Autodesk Fusion 360 part; units mm, degrees
(part 6 of 7)
extrude "v21 socket head clearance (2)" cut sketch "v21 socket head clearance profile (2)" against normal blind 3.22 bodies 1 in component "01 Front optical bezel"
ref_plane "WorkPlane88" through (0, 0, -9.48) normal (0, 0, 1) x (1, 0, 0) in component "05 Rear electronics housing"
sketch "v21 closure blind clearance profile (2)" plane through (0, 0, -9.48) normal (0, 0, 1) x (1, 0, 0) in component "05 Rear electronics housing"
  circle A0 centre (6, 54) radius 1.8
  dimension "d1678" = 3.6
  measures "d1678" diameter of A0
extrude "v21 closure blind clearance (2)" cut sketch "v21 closure blind clearance profile (2)" against normal blind 19.72 bodies 66 in component "05 Rear electronics housing"
ref_plane "WorkPlane67" through (0, 0, 0.02) normal (0, 0, 1) x (1, 0, 0) in component "01 Front optical bezel"
sketch "v21 closure screw clearance profile (3)" plane through (0, 0, 0.02) normal (0, 0, 1) x (1, 0, 0) in component "01 Front optical bezel"
  circle A0 centre (96, 54) radius 1.8
  dimension "d1683" = 3.6
  measures "d1683" diameter of A0
extrude "v21 closure screw clearance (3)" cut sketch "v21 closure screw clearance profile (3)" against normal blind 9.6 bodies 1 in component "01 Front optical bezel"
ref_plane "WorkPlane68" through (0, 0, 0.02) normal (0, 0, 1) x (1, 0, 0) in component "01 Front optical bezel"
sketch "v21 socket head clearance profile (3)" plane through (0, 0, 0.02) normal (0, 0, 1) x (1, 0, 0) in component "01 Front optical bezel"
  circle A0 centre (96, 54) radius 3.4
  dimension "d1688" = 6.8
  measures "d1688" diameter of A0
extrude "v21 socket head clearance (3)" cut sketch "v21 socket head clearance profile (3)" against normal blind 3.22 bodies 1 in component "01 Front optical bezel"
ref_plane "WorkPlane89" through (0, 0, -9.48) normal (0, 0, 1) x (1, 0, 0) in component "05 Rear electronics housing"
sketch "v21 closure blind clearance profile (3)" plane through (0, 0, -9.48) normal (0, 0, 1) x (1, 0, 0) in component "05 Rear electronics housing"
  circle A0 centre (96, 54) radius 1.8
  dimension "d1693" = 3.6
  measures "d1693" diameter of A0
extrude "v21 closure blind clearance (3)" cut sketch "v21 closure blind clearance profile (3)" against normal blind 19.72 bodies 66 in component "05 Rear electronics housing"
ref_plane "WorkPlane69" through (0, 0, -2.6) normal (0, 0, 1) x (1, 0, 0) in component "01 Front optical bezel"
sketch "v21 optical blind clearance profile" plane through (0, 0, -2.6) normal (0, 0, 1) x (1, 0, 0) in component "01 Front optical bezel"
  circle A0 centre (60, 6) radius 1.8
  dimension "d1698" = 3.6
  measures "d1698" diameter of A0
extrude "v21 optical blind clearance" cut sketch "v21 optical blind clearance profile" against normal blind 4.9 bodies 1 in component "01 Front optical bezel"
ref_plane "WorkPlane15" through (0, 0, -7.45) normal (0, 0, 1) x (1, 0, 0) in component "04 Optical retainer"
sketch "v21 optical screw clearance profile" plane through (0, 0, -7.45) normal (0, 0, 1) x (1, 0, 0) in component "04 Optical retainer"
  circle A0 centre (60, 6) radius 1.8
  dimension "d1703" = 3.6
  measures "d1703" diameter of A0
extrude "v21 optical screw clearance" cut sketch "v21 optical screw clearance profile" against normal blind 1.65 bodies 53 in component "04 Optical retainer"
ref_plane "WorkPlane70" through (0, 0, -2.6) normal (0, 0, 1) x (1, 0, 0) in component "01 Front optical bezel"
sketch "v21 optical blind clearance profile (1)" plane through (0, 0, -2.6) normal (0, 0, 1) x (1, 0, 0) in component "01 Front optical bezel"
  circle A0 centre (60, 54) radius 1.8
  dimension "d1708" = 3.6
  measures "d1708" diameter of A0
extrude "v21 optical blind clearance (1)" cut sketch "v21 optical blind clearance profile (1)" against normal blind 4.9 bodies 1 in component "01 Front optical bezel"
ref_plane "WorkPlane16" through (0, 0, -7.45) normal (0, 0, 1) x (1, 0, 0) in component "04 Optical retainer"
sketch "v21 optical screw clearance profile (1)" plane through (0, 0, -7.45) normal (0, 0, 1) x (1, 0, 0) in component "04 Optical retainer"
  circle A0 centre (60, 54) radius 1.8
  dimension "d1713" = 3.6
  measures "d1713" diameter of A0
extrude "v21 optical screw clearance (1)" cut sketch "v21 optical screw clearance profile (1)" against normal blind 1.65 bodies 53 in component "04 Optical retainer"
ref_plane "WorkPlane90" through (0, 0, -11.38) normal (0, 0, 1) x (1, 0, 0) in component "05 Rear electronics housing"
sketch "v21 yoke blind clearance profile" plane through (0, 0, -11.38) normal (0, 0, 1) x (1, 0, 0) in component "05 Rear electronics housing"
  circle A0 centre (35, 38) radius 1.8
  dimension "d1718" = 3.6
  measures "d1718" diameter of A0
extrude "v21 yoke blind clearance" cut sketch "v21 yoke blind clearance profile" against normal blind 6.82 bodies 66 in component "05 Rear electronics housing"
ref_plane "WorkPlane42" through (0, 0, -9.38) normal (0, 0, 1) x (1, 0, 0) in component "06 Electronics retaining yoke"
sketch "v21 yoke screw clearance profile" plane through (0, 0, -9.38) normal (0, 0, 1) x (1, 0, 0) in component "06 Electronics retaining yoke"
  circle A0 centre (35, 38) radius 1.8
  dimension "d1723" = 3.6
  measures "d1723" diameter of A0
extrude "v21 yoke screw clearance" cut sketch "v21 yoke screw clearance profile" against normal blind 2.04 bodies 106 in component "06 Electronics retaining yoke"
ref_plane "WorkPlane91" through (0, 0, -11.38) normal (0, 0, 1) x (1, 0, 0) in component "05 Rear electronics housing"
sketch "v21 yoke blind clearance profile (1)" plane through (0, 0, -11.38) normal (0, 0, 1) x (1, 0, 0) in component "05 Rear electronics housing"
  circle A0 centre (103, 38) radius 1.8
  dimension "d1728" = 3.6
  measures "d1728" diameter of A0
extrude "v21 yoke blind clearance (1)" cut sketch "v21 yoke blind clearance profile (1)" against normal blind 6.82 bodies 66 in component "05 Rear electronics housing"
ref_plane "WorkPlane43" through (0, 0, -9.38) normal (0, 0, 1) x (1, 0, 0) in component "06 Electronics retaining yoke"
sketch "v21 yoke screw clearance profile (1)" plane through (0, 0, -9.38) normal (0, 0, 1) x (1, 0, 0) in component "06 Electronics retaining yoke"
  circle A0 centre (103, 38) radius 1.8
  dimension "d1733" = 3.6
  measures "d1733" diameter of A0
extrude "v21 yoke screw clearance (1)" cut sketch "v21 yoke screw clearance profile (1)" against normal blind 2.04 bodies 106 in component "06 Electronics retaining yoke"
ref_plane "WorkPlane44" through (0, 0, -22.85) normal (0, 0, 1) x (1, 0, 0) in component "06 Electronics retaining yoke"
sketch "v21 PCB axial clearance profile" plane through (0, 0, -22.85) normal (0, 0, 1) x (1, 0, 0) in component "06 Electronics retaining yoke"
  line L0 (13.09, 33.99) -> (15.11, 33.99)
  line L1 (15.11, 33.99) -> (15.11, 36.01)
  line L2 (15.11, 36.01) -> (13.09, 36.01)
  line L3 (13.09, 36.01) -> (13.09, 33.99)
  dimension "d1738" = 2.02
  dimension "d1739" = 2.02
  measures "d1738" horizontal distance of L0.start L0.end
  measures "d1739" vertical distance of L0.end L1.end
extrude "v21 PCB axial clearance" cut sketch "v21 PCB axial clearance profile" against normal blind 0.22 bodies 106 in component "06 Electronics retaining yoke"
ref_plane "WorkPlane45" through (0, 0, -22.85) normal (0, 0, 1) x (1, 0, 0) in component "06 Electronics retaining yoke"
sketch "v21 PCB axial clearance profile (1)" plane through (0, 0, -22.85) normal (0, 0, 1) x (1, 0, 0) in component "06 Electronics retaining yoke"
  line L0 (13.09, 50.99) -> (15.11, 50.99)
  line L1 (15.11, 50.99) -> (15.11, 53.01)
  line L2 (15.11, 53.01) -> (13.09, 53.01)
  line L3 (13.09, 53.01) -> (13.09, 50.99)
  dimension "d1744" = 2.02
  dimension "d1745" = 2.02
  measures "d1744" horizontal distance of L0.start L0.end
  measures "d1745" vertical distance of L0.end L1.end
extrude "v21 PCB axial clearance (1)" cut sketch "v21 PCB axial clearance profile (1)" against normal blind 0.22 bodies 106 in component "06 Electronics retaining yoke"
ref_plane "WorkPlane46" through (0, 0, -22.85) normal (0, 0, 1) x (1, 0, 0) in component "06 Electronics retaining yoke"
sketch "v21 PCB axial clearance profile (2)" plane through (0, 0, -22.85) normal (0, 0, 1) x (1, 0, 0) in component "06 Electronics retaining yoke"
  line L0 (26.89, 33.99) -> (28.91, 33.99)
  line L1 (28.91, 33.99) -> (28.91, 36.01)
  line L2 (28.91, 36.01) -> (26.89, 36.01)
  line L3 (26.89, 36.01) -> (26.89, 33.99)
  dimension "d1750" = 2.02
  dimension "d1751" = 2.02
  measures "d1750" horizontal distance of L0.start L0.end
  measures "d1751" vertical distance of L0.end L1.end
extrude "v21 PCB axial clearance (2)" cut sketch "v21 PCB axial clearance profile (2)" against normal blind 0.22 bodies 106 in component "06 Electronics retaining yoke"
ref_plane "WorkPlane47" through (0, 0, -22.85) normal (0, 0, 1) x (1, 0, 0) in component "06 Electronics retaining yoke"
sketch "v21 PCB axial clearance profile (3)" plane through (0, 0, -22.85) normal (0, 0, 1) x (1, 0, 0) in component "06 Electronics retaining yoke"
  line L0 (26.89, 50.99) -> (28.91, 50.99)
  line L1 (28.91, 50.99) -> (28.91, 53.01)
  line L2 (28.91, 53.01) -> (26.89, 53.01)
  line L3 (26.89, 53.01) -> (26.89, 50.99)
  dimension "d1756" = 2.02
  dimension "d1757" = 2.02
  measures "d1756" horizontal distance of L0.start L0.end
  measures "d1757" vertical distance of L0.end L1.end
extrude "v21 PCB axial clearance (3)" cut sketch "v21 PCB axial clearance profile (3)" against normal blind 0.22 bodies 106 in component "06 Electronics retaining yoke"
ref_plane "WorkPlane48" through (0, 0, -19.65) normal (0, 0, 1) x (1, 0, 0) in component "06 Electronics retaining yoke"
sketch "v21 DPDT axial clearance profile" plane through (0, 0, -19.65) normal (0, 0, 1) x (1, 0, 0) in component "06 Electronics retaining yoke"
  line L0 (55.89, 49.69) -> (56.91, 49.69)
  line L1 (56.91, 49.69) -> (56.91, 52.01)
  line L2 (56.91, 52.01) -> (55.89, 52.01)
  line L3 (55.89, 52.01) -> (55.89, 49.69)
  dimension "d1762" = 1.02
  dimension "d1763" = 2.32
  measures "d1762" horizontal distance of L0.start L0.end
  measures "d1763" vertical distance of L0.end L1.end
extrude "v21 DPDT axial clearance" cut sketch "v21 DPDT axial clearance profile" against normal blind 0.22 bodies 106 in component "06 Electronics retaining yoke"
ref_plane "WorkPlane49" through (0, 0, -19.65) normal (0, 0, 1) x (1, 0, 0) in component "06 Electronics retaining yoke"
sketch "v21 DPDT axial clearance profile (1)" plane through (0, 0, -19.65) normal (0, 0, 1) x (1, 0, 0) in component "06 Electronics retaining yoke"
  line L0 (63.09, 49.69) -> (64.11, 49.69)
  line L1 (64.11, 49.69) -> (64.11, 52.01)
  line L2 (64.11, 52.01) -> (63.09, 52.01)
  line L3 (63.09, 52.01) -> (63.09, 49.69)
  dimension "d1768" = 1.02
  dimension "d1769" = 2.32
  measures "d1768" horizontal distance of L0.start L0.end
  measures "d1769" vertical distance of L0.end L1.end
extrude "v21 DPDT axial clearance (1)" cut sketch "v21 DPDT axial clearance profile (1)" against normal blind 0.22 bodies 106 in component "06 Electronics retaining yoke"
ref_plane "WorkPlane50" through (0, 0, -11.2) normal (0, 0, 1) x (1, 0, 0) in component "06 Electronics retaining yoke"
sketch "v21 XIAO axial clearance profile" plane through (0, 0, -11.2) normal (0, 0, 1) x (1, 0, 0) in component "06 Electronics retaining yoke"
  line L0 (110.8, 35.4) -> (112.1, 35.4)
  line L1 (112.1, 35.4) -> (112.1, 56.6)
  line L2 (112.1, 56.6) -> (110.8, 56.6)
  line L3 (110.8, 56.6) -> (110.8, 35.4)
  dimension "d1774" = 1.3
  dimension "d1775" = 21.2
  measures "d1774" horizontal distance of L0.start L0.end
  measures "d1775" vertical distance of L0.end L1.end
extrude "v21 XIAO axial clearance" cut sketch "v21 XIAO axial clearance profile" against normal blind 0.25 bodies 106 in component "06 Electronics retaining yoke"
ref_plane "WorkPlane17" through (0, 0, -7.47) normal (0, 0, 1) x (1, 0, 0) in component "04 Optical retainer"
sketch "v21 optical stack allowance profile" plane through (0, 0, -7.47) normal (0, 0, 1) x (1, 0, 0) in component "04 Optical retainer"
  line L0 (7.99, 10.99) -> (112.01, 10.99)
  line L1 (112.01, 10.99) -> (112.01, 49.01)
  line L2 (112.01, 49.01) -> (7.99, 49.01)
  line L3 (7.99, 49.01) -> (7.99, 10.99)
  dimension "d1780" = 104.02
  dimension "d1781" = 38.02
  measures "d1780" horizontal distance of L0.start L0.end
  measures "d1781" vertical distance of L0.end L1.end
extrude "v21 optical stack allowance" cut sketch "v21 optical stack allowance profile" against normal blind 0.255 bodies 53 in component "04 Optical retainer"
ref_plane "WorkPlane18" through (0, 0, -4.34) normal (0, 0, 1) x (1, 0, 0) in component "04 Optical retainer"
sketch "v21 LED cushion clearance profile" plane through (0, 0, -4.34) normal (0, 0, 1) x (1, 0, 0) in component "04 Optical retainer"
  line L0 (38.49, 5.19) -> (41.51, 5.19)
  line L1 (41.51, 5.19) -> (41.51, 10.81)
  line L2 (41.51, 10.81) -> (38.49, 10.81)
  line L3 (38.49, 10.81) -> (38.49, 5.19)
  dimension "d1786" = 3.02
  dimension "d1787" = 5.62
  measures "d1786" horizontal distance of L0.start L0.end
  measures "d1787" vertical distance of L0.end L1.end
extrude "v21 LED cushion clearance" cut sketch "v21 LED cushion clearance profile" against normal blind 0.26 bodies 53 in component "04 Optical retainer"
ref_plane "WorkPlane19" through (0, 0, -4.34) normal (0, 0, 1) x (1, 0, 0) in component "04 Optical retainer"
sketch "v21 LED cushion clearance profile (1)" plane through (0, 0, -4.34) normal (0, 0, 1) x (1, 0, 0) in component "04 Optical retainer"
  line L0 (38.49, 49.19) -> (41.51, 49.19)
  line L1 (41.51, 49.19) -> (41.51, 54.81)
  line L2 (41.51, 54.81) -> (38.49, 54.81)
  line L3 (38.49, 54.81) -> (38.49, 49.19)
  dimension "d1792" = 3.02
  dimension "d1793" = 5.62
  measures "d1792" horizontal distance of L0.start L0.end
  measures "d1793" vertical distance of L0.end L1.end
extrude "v21 LED cushion clearance (1)" cut sketch "v21 LED cushion clearance profile (1)" against normal blind 0.26 bodies 53 in component "04 Optical retainer"
ref_plane "WorkPlane20" through (0, 0, -4.34) normal (0, 0, 1) x (1, 0, 0) in component "04 Optical retainer"
sketch "v21 LED cushion clearance profile (2)" plane through (0, 0, -4.34) normal (0, 0, 1) x (1, 0, 0) in component "04 Optical retainer"
  line L0 (78.49, 5.19) -> (81.51, 5.19)
  line L1 (81.51, 5.19) -> (81.51, 10.81)
  line L2 (81.51, 10.81) -> (78.49, 10.81)
  line L3 (78.49, 10.81) -> (78.49, 5.19)
  dimension "d1798" = 3.02
  dimension "d1799" = 5.62
  measures "d1798" horizontal distance of L0.start L0.end
  measures "d1799" vertical distance of L0.end L1.end
extrude "v21 LED cushion clearance (2)" cut sketch "v21 LED cushion clearance profile (2)" against normal blind 0.26 bodies 53 in component "04 Optical retainer"
ref_plane "WorkPlane21" through (0, 0, -4.34) normal (0, 0, 1) x (1, 0, 0) in component "04 Optical retainer"
sketch "v21 LED cushion clearance profile (3)" plane through (0, 0, -4.34) normal (0, 0, 1) x (1, 0, 0) in component "04 Optical retainer"
  line L0 (78.49, 49.19) -> (81.51, 49.19)
  line L1 (81.51, 49.19) -> (81.51, 54.81)
  line L2 (81.51, 54.81) -> (78.49, 54.81)
  line L3 (78.49, 54.81) -> (78.49, 49.19)
  dimension "d1804" = 3.02
  dimension "d1805" = 5.62
  measures "d1804" horizontal distance of L0.start L0.end
  measures "d1805" vertical distance of L0.end L1.end
extrude "v21 LED cushion clearance (3)" cut sketch "v21 LED cushion clearance profile (3)" against normal blind 0.26 bodies 53 in component "04 Optical retainer"
ref_plane "WorkPlane71" through (0, 0, -2.4) normal (0, 0, 1) x (1, 0, 0) in component "01 Front optical bezel"
sketch "v21 LED solder-wire exit profile" plane through (0, 0, -2.4) normal (0, 0, 1) x (1, 0, 0) in component "01 Front optical bezel"
  line L0 (34.4, 4.8) -> (35.9, 4.8)
  line L1 (35.9, 4.8) -> (35.9, 8.8)
  line L2 (35.9, 8.8) -> (34.4, 8.8)
  line L3 (34.4, 8.8) -> (34.4, 4.8)
  dimension "d1810" = 1.5
  dimension "d1811" = 4
  measures "d1810" horizontal distance of L0.start L0.end
  measures "d1811" vertical distance of L0.end L1.end
extrude "v21 LED solder-wire exit" cut sketch "v21 LED solder-wire exit profile" against normal blind 2.2 bodies 1 in component "01 Front optical bezel"
ref_plane "WorkPlane72" through (0, 0, -2.4) normal (0, 0, 1) x (1, 0, 0) in component "01 Front optical bezel"
sketch "v21 LED solder-wire exit profile (1)" plane through (0, 0, -2.4) normal (0, 0, 1) x (1, 0, 0) in component "01 Front optical bezel"
  line L0 (44.1, 4.8) -> (45.6, 4.8)
  line L1 (45.6, 4.8) -> (45.6, 8.8)
  line L2 (45.6, 8.8) -> (44.1, 8.8)
  line L3 (44.1, 8.8) -> (44.1, 4.8)
  dimension "d1816" = 1.5
  dimension "d1817" = 4
  measures "d1816" horizontal distance of L0.start L0.end
  measures "d1817" vertical distance of L0.end L1.end
extrude "v21 LED solder-wire exit (1)" cut sketch "v21 LED solder-wire exit profile (1)" against normal blind 2.2 bodies 1 in component "01 Front optical bezel"
ref_plane "WorkPlane73" through (0, 0, -2.4) normal (0, 0, 1) x (1, 0, 0) in component "01 Front optical bezel"
sketch "v21 LED solder-wire exit profile (2)" plane through (0, 0, -2.4) normal (0, 0, 1) x (1, 0, 0) in component "01 Front optical bezel"
  line L0 (34.4, 51.2) -> (35.9, 51.2)
  line L1 (35.9, 51.2) -> (35.9, 55.2)
  line L2 (35.9, 55.2) -> (34.4, 55.2)
  line L3 (34.4, 55.2) -> (34.4, 51.2)
  dimension "d1822" = 1.5
  dimension "d1823" = 4
  measures "d1822" horizontal distance of L0.start L0.end
  measures "d1823" vertical distance of L0.end L1.end
extrude "v21 LED solder-wire exit (2)" cut sketch "v21 LED solder-wire exit profile (2)" against normal blind 2.2 bodies 1 in component "01 Front optical bezel"
ref_plane "WorkPlane74" through (0, 0, -2.4) normal (0, 0, 1) x (1, 0, 0) in component "01 Front optical bezel"
sketch "v21 LED solder-wire exit profile (3)" plane through (0, 0, -2.4) normal (0, 0, 1) x (1, 0, 0) in component "01 Front optical bezel"
  line L0 (44.1, 51.2) -> (45.6, 51.2)
  line L1 (45.6, 51.2) -> (45.6, 55.2)
  line L2 (45.6, 55.2) -> (44.1, 55.2)
  line L3 (44.1, 55.2) -> (44.1, 51.2)
  dimension "d1828" = 1.5
  dimension "d1829" = 4
  measures "d1828" horizontal distance of L0.start L0.end
  measures "d1829" vertical distance of L0.end L1.end
extrude "v21 LED solder-wire exit (3)" cut sketch "v21 LED solder-wire exit profile (3)" against normal blind 2.2 bodies 1 in component "01 Front optical bezel"
ref_plane "WorkPlane75" through (0, 0, -2.4) normal (0, 0, 1) x (1, 0, 0) in component "01 Front optical bezel"
sketch "v21 LED solder-wire exit profile (4)" plane through (0, 0, -2.4) normal (0, 0, 1) x (1, 0, 0) in component "01 Front optical bezel"
  line L0 (74.4, 4.8) -> (75.9, 4.8)
  line L1 (75.9, 4.8) -> (75.9, 8.8)
  line L2 (75.9, 8.8) -> (74.4, 8.8)
  line L3 (74.4, 8.8) -> (74.4, 4.8)
  dimension "d1834" = 1.5
  dimension "d1835" = 4
  measures "d1834" horizontal distance of L0.start L0.end
  measures "d1835" vertical distance of L0.end L1.end
extrude "v21 LED solder-wire exit (4)" cut sketch "v21 LED solder-wire exit profile (4)" against normal blind 2.2 bodies 1 in component "01 Front optical bezel"
ref_plane "WorkPlane76" through (0, 0, -2.4) normal (0, 0, 1) x (1, 0, 0) in component "01 Front optical bezel"
sketch "v21 LED solder-wire exit profile (5)" plane through (0, 0, -2.4) normal (0, 0, 1) x (1, 0, 0) in component "01 Front optical bezel"
  line L0 (84.1, 4.8) -> (85.6, 4.8)
  line L1 (85.6, 4.8) -> (85.6, 8.8)
  line L2 (85.6, 8.8) -> (84.1, 8.8)
  line L3 (84.1, 8.8) -> (84.1, 4.8)
  dimension "d1840" = 1.5
  dimension "d1841" = 4
  measures "d1840" horizontal distance of L0.start L0.end
  measures "d1841" vertical distance of L0.end L1.end
extrude "v21 LED solder-wire exit (5)" cut sketch "v21 LED solder-wire exit profile (5)" against normal blind 2.2 bodies 1 in component "01 Front optical bezel"
ref_plane "WorkPlane77" through (0, 0, -2.4) normal (0, 0, 1) x (1, 0, 0) in component "01 Front optical bezel"
sketch "v21 LED solder-wire exit profile (6)" plane through (0, 0, -2.4) normal (0, 0, 1) x (1, 0, 0) in component "01 Front optical bezel"
  line L0 (74.4, 51.2) -> (75.9, 51.2)
  line L1 (75.9, 51.2) -> (75.9, 55.2)
  line L2 (75.9, 55.2) -> (74.4, 55.2)
  line L3 (74.4, 55.2) -> (74.4, 51.2)
  dimension "d1846" = 1.5
  dimension "d1847" = 4
  measures "d1846" horizontal distance of L0.start L0.end
  measures "d1847" vertical distance of L0.end L1.end
extrude "v21 LED solder-wire exit (6)" cut sketch "v21 LED solder-wire exit profile (6)" against normal blind 2.2 bodies 1 in component "01 Front optical bezel"
ref_plane "WorkPlane78" through (0, 0, -2.4) normal (0, 0, 1) x (1, 0, 0) in component "01 Front optical bezel"
sketch "v21 LED solder-wire exit profile (7)" plane through (0, 0, -2.4) normal (0, 0, 1) x (1, 0, 0) in component "01 Front optical bezel"
  line L0 (84.1, 51.2) -> (85.6, 51.2)
  line L1 (85.6, 51.2) -> (85.6, 55.2)
  line L2 (85.6, 55.2) -> (84.1, 55.2)
  line L3 (84.1, 55.2) -> (84.1, 51.2)
  dimension "d1852" = 1.5
  dimension "d1853" = 4
  measures "d1852" horizontal distance of L0.start L0.end
  measures "d1853" vertical distance of L0.end L1.end
extrude "v21 LED solder-wire exit (7)" cut sketch "v21 LED solder-wire exit profile (7)" against normal blind 2.2 bodies 1 in component "01 Front optical bezel"
ref_plane "WorkPlane8" through (0, 0, -18) normal (0, 0, 1) x (1, 0, 0) in component "08 Captive RUN PROGRAM slider"
sketch "v21 actuator running clearance profile" plane through (0, 0, -18) normal (0, 0, 1) x (1, 0, 0) in component "08 Captive RUN PROGRAM slider"
  line L0 (58.95, 52.3) -> (61.05, 52.3)
  line L1 (61.05, 52.3) -> (61.05, 54.53)
  line L2 (61.05, 54.53) -> (58.95, 54.53)
  line L3 (58.95, 54.53) -> (58.95, 52.3)
  dimension "d1858" = 2.1
  dimension "d1859" = 2.23
  measures "d1858" horizontal distance of L0.start L0.end
  measures "d1859" vertical distance of L0.end L1.end
extrude "v21 actuator running clearance" cut sketch "v21 actuator running clearance profile" against normal blind 4.6 bodies 131 in component "08 Captive RUN PROGRAM slider"
ref_plane "WorkPlane92" through (0, 0, -13.6) normal (0, 0, 1) x (1, 0, 0) in component "05 Rear electronics housing"
sketch "v21 reset guide running clearance profile" plane through (0, 0, -13.6) normal (0, 0, 1) x (1, 0, 0) in component "05 Rear electronics housing"
  line L0 (116.1, 52.45) -> (120.2, 52.45)
  line L1 (120.2, 52.45) -> (120.2, 56.95)
  line L2 (120.2, 56.95) -> (116.1, 56.95)
  line L3 (116.1, 56.95) -> (116.1, 52.45)
  dimension "d1864" = 4.1
  dimension "d1865" = 4.5
  measures "d1864" horizontal distance of L0.start L0.end
  measures "d1865" vertical distance of L0.end L1.end
extrude "v21 reset guide running clearance" cut sketch "v21 reset guide running clearance profile" against normal blind 3.1 bodies 66 in component "05 Rear electronics housing"
ref_plane "WorkPlane51" through (0, 0, -13.6) normal (0, 0, 1) x (1, 0, 0) in component "06 Electronics retaining yoke"
sketch "v21 reset roof running clearance profile" plane through (0, 0, -13.6) normal (0, 0, 1) x (1, 0, 0) in component "06 Electronics retaining yoke"
  line L0 (116.19, 52.79) -> (119.76, 52.79)
  line L1 (119.76, 52.79) -> (119.76, 56.61)
  line L2 (119.76, 56.61) -> (116.19, 56.61)
  line L3 (116.19, 56.61) -> (116.19, 52.79)
  dimension "d1870" = 3.57
  dimension "d1871" = 3.82
  measures "d1870" horizontal distance of L0.start L0.end
  measures "d1871" vertical distance of L0.end L1.end
extrude "v21 reset roof running clearance" cut sketch "v21 reset roof running clearance profile" against normal blind 0.12 bodies 106 in component "06 Electronics retaining yoke"
ref_plane "WorkPlane93" through (0, 0, -29.5) normal (0, 0, 1) x (1, 0, 0) in component "05 Rear electronics housing"
sketch "BOOST insulating landing profile" plane through (0, 0, -29.5) normal (0, 0, 1) x (1, 0, 0) in component "05 Rear electronics housing"
  line L0 (37, 41.5) -> (52.3, 41.5)
  line L1 (52.3, 41.5) -> (52.3, 52.5)
  line L2 (52.3, 52.5) -> (37, 52.5)
  line L3 (37, 52.5) -> (37, 41.5)
  dimension "d1876" = 15.3
  dimension "d1877" = 11
  measures "d1876" horizontal distance of L0.start L0.end
  measures "d1877" vertical distance of L0.end L1.end
extrude "BOOST insulating landing" add sketch "BOOST insulating landing profile" against normal blind 2.2 separate body makes body 197 in component "05 Rear electronics housing"
ref_plane "WorkPlane94" through (0, 0, -27.5) normal (0, 0, 1) x (1, 0, 0) in component "05 Rear electronics housing"
sketch "BOOST lateral locating fence profile" plane through (0, 0, -27.5) normal (0, 0, 1) x (1, 0, 0) in component "05 Rear electronics housing"
  line L0 (36.1, 41.5) -> (37.3, 41.5)
  line L1 (37.3, 41.5) -> (37.3, 52.5)
  line L2 (37.3, 52.5) -> (36.1, 52.5)
  line L3 (36.1, 52.5) -> (36.1, 41.5)
  dimension "d1882" = 1.2
  dimension "d1883" = 11
  measures "d1882" horizontal distance of L0.start L0.end
  measures "d1883" vertical distance of L0.end L1.end
extrude "BOOST lateral locating fence" add sketch "BOOST lateral locating fence profile" against normal blind 4.2 separate body makes body 198 in component "05 Rear electronics housing"
ref_plane "WorkPlane95" through (0, 0, -27.5) normal (0, 0, 1) x (1, 0, 0) in component "05 Rear electronics housing"
sketch "BOOST lateral locating fence profile (1)" plane through (0, 0, -27.5) normal (0, 0, 1) x (1, 0, 0) in component "05 Rear electronics housing"
  line L0 (52, 41.5) -> (53.2, 41.5)
  line L1 (53.2, 41.5) -> (53.2, 52.5)
  line L2 (53.2, 52.5) -> (52, 52.5)
  line L3 (52, 52.5) -> (52, 41.5)
  dimension "d1888" = 1.2
  dimension "d1889" = 11
  measures "d1888" horizontal distance of L0.start L0.end
  measures "d1889" vertical distance of L0.end L1.end
extrude "BOOST lateral locating fence (1)" add sketch "BOOST lateral locating fence profile (1)" against normal blind 4.2 separate body makes body 199 in component "05 Rear electronics housing"
ref_plane "WorkPlane96" through (0, 0, -29.5) normal (0, 0, 1) x (1, 0, 0) in component "05 Rear electronics housing"
sketch "SIGNAL insulating landing profile" plane through (0, 0, -29.5) normal (0, 0, 1) x (1, 0, 0) in component "05 Rear electronics housing"
  line L0 (71, 41) -> (90.5, 41)
  line L1 (90.5, 41) -> (90.5, 53.5)
  line L2 (90.5, 53.5) -> (71, 53.5)
  line L3 (71, 53.5) -> (71, 41)
  dimension "d1894" = 19.5
  dimension "d1895" = 12.5
  measures "d1894" horizontal distance of L0.start L0.end
  measures "d1895" vertical distance of L0.end L1.end
extrude "SIGNAL insulating landing" add sketch "SIGNAL insulating landing profile" against normal blind 2.2 separate body makes body 200 in component "05 Rear electronics housing"
ref_plane "WorkPlane97" through (0, 0, -27.5) normal (0, 0, 1) x (1, 0, 0) in component "05 Rear electronics housing"
sketch "SIGNAL lateral locating fence profile" plane through (0, 0, -27.5) normal (0, 0, 1) x (1, 0, 0) in component "05 Rear electronics housing"
  line L0 (70.1, 41) -> (71.3, 41)
  line L1 (71.3, 41) -> (71.3, 53.5)
  line L2 (71.3, 53.5) -> (70.1, 53.5)
  line L3 (70.1, 53.5) -> (70.1, 41)
  dimension "d1900" = 1.2
  dimension "d1901" = 12.5
  measures "d1900" horizontal distance of L0.start L0.end
  measures "d1901" vertical distance of L0.end L1.end
extrude "SIGNAL lateral locating fence" add sketch "SIGNAL lateral locating fence profile" against normal blind 4.2 separate body makes body 201 in component "05 Rear electronics housing"
ref_plane "WorkPlane98" through (0, 0, -27.5) normal (0, 0, 1) x (1, 0, 0) in component "05 Rear electronics housing"
sketch "SIGNAL lateral locating fence profile (1)" plane through (0, 0, -27.5) normal (0, 0, 1) x (1, 0, 0) in component "05 Rear electronics housing"
  line L0 (90.2, 41) -> (91.4, 41)
  line L1 (91.4, 41) -> (91.4, 53.5)
  line L2 (91.4, 53.5) -> (90.2, 53.5)
  line L3 (90.2, 53.5) -> (90.2, 41)
  dimension "d1906" = 1.2
  dimension "d1907" = 12.5
  measures "d1906" horizontal distance of L0.start L0.end
  measures "d1907" vertical distance of L0.end L1.end
extrude "SIGNAL lateral locating fence (1)" add sketch "SIGNAL lateral locating fence profile (1)" against normal blind 4.2 separate body makes body 202 in component "05 Rear electronics housing"
ref_plane "WorkPlane99" through (0, 0, -22) normal (0, 0, 1) x (1, 0, 0) in component "05 Rear electronics housing"
sketch "Harness strap anchor profile" plane through (0, 0, -22) normal (0, 0, 1) x (1, 0, 0) in component "05 Rear electronics housing"
  line L0 (14, 14.5) -> (20, 14.5)
  line L1 (20, 14.5) -> (20, 21.5)
  line L2 (20, 21.5) -> (14, 21.5)
  line L3 (14, 21.5) -> (14, 14.5)
  dimension "d1912" = 6
  dimension "d1913" = 7
  measures "d1912" horizontal distance of L0.start L0.end
  measures "d1913" vertical distance of L0.end L1.end
extrude "Harness strap anchor" add sketch "Harness strap anchor profile" against normal blind 9.7 separate body makes body 203 in component "05 Rear electronics housing"
ref_plane "WorkPlane100" through (0, 0, -22) normal (0, 0, 1) x (1, 0, 0) in component "05 Rear electronics housing"
sketch "Harness strap anchor profile (1)" plane through (0, 0, -22) normal (0, 0, 1) x (1, 0, 0) in component "05 Rear electronics housing"
  line L0 (96, 16.5) -> (102, 16.5)
  line L1 (102, 16.5) -> (102, 23.5)
  line L2 (102, 23.5) -> (96, 23.5)
  line L3 (96, 23.5) -> (96, 16.5)
  dimension "d1918" = 6
  dimension "d1919" = 7
  measures "d1918" horizontal distance of L0.start L0.end
  measures "d1919" vertical distance of L0.end L1.end
extrude "Harness strap anchor (1)" add sketch "Harness strap anchor profile (1)" against normal blind 9.7 separate body makes body 204 in component "05 Rear electronics housing"
combine "Union manufactured solid (10)" operation add target body 66 tool bodies 197 198 199 200 201 202 203 204 in component "05 Rear electronics housing"
ref_plane "WorkPlane101" through (13.9, 0, 0) normal (1, 0, 0) x (0, 1, 0) in component "05 Rear electronics housing"
sketch "Harness strap passage" plane through (13.9, 0, 0) normal (1, 0, 0) x (0, 0, -1) in component "05 Rear electronics housing"
  line L0 (28.5, 16.5) -> (28.5, 19.5)
  line L1 (28.5, 19.5) -> (25.8, 19.5)
  line L2 (25.8, 19.5) -> (24.3, 18)
  line L3 (24.3, 18) -> (25.8, 16.5)
  line L4 (25.8, 16.5) -> (28.5, 16.5)
extrude "Harness strap passage (1)" cut sketch "Harness strap passage" along normal blind 6.2 bodies 66 in component "05 Rear electronics housing"
ref_plane "WorkPlane102" through (95.9, 0, 0) normal (1, 0, 0) x (0, 1, 0) in component "05 Rear electronics housing"
sketch "Harness strap passage (1)" plane through (95.9, 0, 0) normal (1, 0, 0) x (0, 0, -1) in component "05 Rear electronics housing"
  line L0 (28.5, 18.5) -> (28.5, 21.5)
  line L1 (28.5, 21.5) -> (25.8, 21.5)
  line L2 (25.8, 21.5) -> (24.3, 20)
  line L3 (24.3, 20) -> (25.8, 18.5)
  line L4 (25.8, 18.5) -> (28.5, 18.5)
extrude "Harness strap passage (2)" cut sketch "Harness strap passage (1)" along normal blind 6.2 bodies 66 in component "05 Rear electronics housing"
ref_plane "WorkPlane103" through (0, 0, -11.38) normal (0, 0, 1) x (1, 0, 0) in component "05 Rear electronics housing"
sketch "XIAO underside battery and GPIO solder access profile" plane through (0, 0, -11.38) normal (0, 0, 1) x (1, 0, 0) in component "05 Rear electronics housing"
  line L0 (108.8, 36.8) -> (110.95, 36.8)
  line L1 (110.95, 36.8) -> (110.95, 54.5)
  line L2 (110.95, 54.5) -> (108.8, 54.5)
  line L3 (108.8, 54.5) -> (108.8, 36.8)
  dimension "d1932" = 2.15
  dimension "d1933" = 17.7
  measures "d1932" horizontal distance of L0.start L0.end
  measures "d1933" vertical distance of L0.end L1.end
extrude "XIAO underside battery and GPIO solder access" cut sketch "XIAO underside battery and GPIO solder access profile" against normal blind 17.72 bodies 66 in component "05 Rear electronics housing"
ref_plane "WorkPlane104" through (0, 0, -27.45) normal (0, 0, 1) x (1, 0, 0) in component "05 Rear electronics housing"
sketch "v22 clear unused booster land and fences profile" plane through (0, 0, -27.45) normal (0, 0, 1) x (1, 0, 0) in component "05 Rear electronics housing"
  line L0 (36.05, 41.45) -> (53.25, 41.45)
  line L1 (53.25, 41.45) -> (53.25, 52.55)
  line L2 (53.25, 52.55) -> (36.05, 52.55)
  line L3 (36.05, 52.55) -> (36.05, 41.45)
  dimension "d1969" = 17.2
  dimension "d1970" = 11.1
  measures "d1969" horizontal distance of L0.start L0.end
  measures "d1970" vertical distance of L0.end L1.end
extrude "v22 clear unused booster land and fences" cut sketch "v22 clear unused booster land and fences profile" against normal blind 4.15 bodies 66 in component "05 Rear electronics housing"
ref_plane "WorkPlane105" through (0, 0, -25.7) normal (0, 0, 1) x (1, 0, 0) in component "05 Rear electronics housing"
sketch "SPDT rear seat profile" plane through (0, 0, -25.7) normal (0, 0, 1) x (1, 0, 0) in component "05 Rear electronics housing"
  line L0 (35.45, 51.2) -> (46.55, 51.2)
  line L1 (46.55, 51.2) -> (46.55, 57.35)
  line L2 (46.55, 57.35) -> (35.45, 57.35)
  line L3 (35.45, 57.35) -> (35.45, 51.2)
  dimension "d1975" = 11.1
  dimension "d1976" = 6.15
  measures "d1975" horizontal distance of L0.start L0.end
  measures "d1976" vertical distance of L0.end L1.end
extrude "SPDT rear seat" add sketch "SPDT rear seat profile" against normal blind 6 separate body makes body 205 in component "05 Rear electronics housing"
ref_plane "WorkPlane106" through (0, 0, -19.8) normal (0, 0, 1) x (1, 0, 0) in component "05 Rear electronics housing"
sketch "SPDT side locating cheek profile" plane through (0, 0, -19.8) normal (0, 0, 1) x (1, 0, 0) in component "05 Rear electronics housing"
  line L0 (34.05, 51.2) -> (35.45, 51.2)
  line L1 (35.45, 51.2) -> (35.45, 56.25)
  line L2 (35.45, 56.25) -> (34.05, 56.25)
  line L3 (34.05, 56.25) -> (34.05, 51.2)
  dimension "d1981" = 1.4
  dimension "d1982" = 5.05
  measures "d1981" horizontal distance of L0.start L0.end
  measures "d1982" vertical distance of L0.end L1.end
extrude "SPDT side locating cheek" add sketch "SPDT side locating cheek profile" against normal blind 11.9 separate body makes body 206 in component "05 Rear electronics housing"
ref_plane "WorkPlane107" through (0, 0, -19.8) normal (0, 0, 1) x (1, 0, 0) in component "05 Rear electronics housing"
sketch "SPDT side locating cheek profile (1)" plane through (0, 0, -19.8) normal (0, 0, 1) x (1, 0, 0) in component "05 Rear electronics housing"
  line L0 (46.55, 51.2) -> (47.95, 51.2)
  line L1 (47.95, 51.2) -> (47.95, 56.25)
  line L2 (47.95, 56.25) -> (46.55, 56.25)
  line L3 (46.55, 56.25) -> (46.55, 51.2)
  dimension "d1987" = 1.4
  dimension "d1988" = 5.05
  measures "d1987" horizontal distance of L0.start L0.end
  measures "d1988" vertical distance of L0.end L1.end
extrude "SPDT side locating cheek (1)" add sketch "SPDT side locating cheek profile (1)" against normal blind 11.9 separate body makes body 207 in component "05 Rear electronics housing"
ref_plane "WorkPlane108" through (0, 0, -20) normal (0, 0, 1) x (1, 0, 0) in component "05 Rear electronics housing"
sketch "SPDT terminal-side shoulder stop profile" plane through (0, 0, -20) normal (0, 0, 1) x (1, 0, 0) in component "05 Rear electronics housing"
  line L0 (35.45, 49.9) -> (36.45, 49.9)
  line L1 (36.45, 49.9) -> (36.45, 51.2)
  line L2 (36.45, 51.2) -> (35.45, 51.2)
  line L3 (35.45, 51.2) -> (35.45, 49.9)
  dimension "d1993" = 1
  dimension "d1994" = 1.3
  measures "d1993" horizontal distance of L0.start L0.end
  measures "d1994" vertical distance of L0.end L1.end
extrude "SPDT terminal-side shoulder stop" add sketch "SPDT terminal-side shoulder stop profile" against normal blind 11.7 separate body makes body 208 in component "05 Rear electronics housing"
ref_plane "WorkPlane109" through (0, 0, -20) normal (0, 0, 1) x (1, 0, 0) in component "05 Rear electronics housing"
sketch "SPDT terminal-side shoulder stop profile (1)" plane through (0, 0, -20) normal (0, 0, 1) x (1, 0, 0) in component "05 Rear electronics housing"
  line L0 (45.55, 49.9) -> (46.55, 49.9)
  line L1 (46.55, 49.9) -> (46.55, 51.2)
  line L2 (46.55, 51.2) -> (45.55, 51.2)
  line L3 (45.55, 51.2) -> (45.55, 49.9)
  dimension "d1999" = 1
  dimension "d2000" = 1.3
  measures "d1999" horizontal distance of L0.start L0.end
  measures "d2000" vertical distance of L0.end L1.end
extrude "SPDT terminal-side shoulder stop (1)" add sketch "SPDT terminal-side shoulder stop profile (1)" against normal blind 11.7 separate body makes body 209 in component "05 Rear electronics housing"
ref_plane "WorkPlane110" through (0, 0, -20) normal (0, 0, 1) x (1, 0, 0) in component "05 Rear electronics housing"
sketch "SPDT flange-side stop tied to top wall profile" plane through (0, 0, -20) normal (0, 0, 1) x (1, 0, 0) in component "05 Rear electronics housing"
  line L0 (35.45, 57.3) -> (46.55, 57.3)
  line L1 (46.55, 57.3) -> (46.55, 57.7)
  line L2 (46.55, 57.7) -> (35.45, 57.7)
  line L3 (35.45, 57.7) -> (35.45, 57.3)
  dimension "d2005" = 11.1
  dimension "d2006" = 0.4
  measures "d2005" horizontal distance of L0.start L0.end
  measures "d2006" vertical distance of L0.end L1.end
extrude "SPDT flange-side stop tied to top wall" add sketch "SPDT flange-side stop tied to top wall profile" against normal blind 11.7 separate body makes body 210 in component "05 Rear electronics housing"
combine "Union manufactured solid (11)" operation add target body 66 tool bodies 205 206 207 208 209 210 in component "05 Rear electronics housing"
ref_plane "WorkPlane111" through (0, 0, -9.45) normal (0, 0, 1) x (1, 0, 0) in component "05 Rear electronics housing"
sketch "SPDT front-loading lever notch profile" plane through (0, 0, -9.45) normal (0, 0, 1) x (1, 0, 0) in component "05 Rear electronics housing"
  line L0 (37.05, 57.25) -> (44.95, 57.25)
  line L1 (44.95, 57.25) -> (44.95, 60.15)
  line L2 (44.95, 60.15) -> (37.05, 60.15)
  line L3 (37.05, 60.15) -> (37.05, 57.25)
  dimension "d2011" = 7.9
  dimension "d2012" = 2.9
  measures "d2011" horizontal distance of L0.start L0.end
  measures "d2012" vertical distance of L0.end L1.end
extrude "SPDT front-loading lever notch" cut sketch "SPDT front-loading lever notch profile" against normal blind 15.35 bodies 66 in component "05 Rear electronics housing"
ref_plane "WorkPlane52" through (0, 0, -9.4) normal (0, 0, 1) x (1, 0, 0) in component "06 Electronics retaining yoke"
sketch "SPDT keeper arm profile" plane through (0, 0, -9.4) normal (0, 0, 1) x (1, 0, 0) in component "06 Electronics retaining yoke"
  line L0 (37.4, 37.5) -> (39.8, 37.5)
  line L1 (39.8, 37.5) -> (39.8, 54.5)
  line L2 (39.8, 54.5) -> (37.4, 54.5)
  line L3 (37.4, 54.5) -> (37.4, 37.5)
  dimension "d2017" = 2.4
  dimension "d2018" = 17
  measures "d2017" horizontal distance of L0.start L0.end
  measures "d2018" vertical distance of L0.end L1.end
extrude "SPDT keeper arm" add sketch "SPDT keeper arm profile" against normal blind 2 separate body makes body 211 in component "06 Electronics retaining yoke"
ref_plane "WorkPlane53" through (0, 0, -9.4) normal (0, 0, 1) x (1, 0, 0) in component "06 Electronics retaining yoke"
sketch "SPDT keeper arm profile (1)" plane through (0, 0, -9.4) normal (0, 0, 1) x (1, 0, 0) in component "06 Electronics retaining yoke"
  line L0 (43.6, 37.5) -> (46, 37.5)
  line L1 (46, 37.5) -> (46, 54.5)
  line L2 (46, 54.5) -> (43.6, 54.5)
  line L3 (43.6, 54.5) -> (43.6, 37.5)
  dimension "d2023" = 2.4
  dimension "d2024" = 17
  measures "d2023" horizontal distance of L0.start L0.end
  measures "d2024" vertical distance of L0.end L1.end
extrude "SPDT keeper arm (1)" add sketch "SPDT keeper arm profile (1)" against normal blind 2 separate body makes body 212 in component "06 Electronics retaining yoke"
ref_plane "WorkPlane54" through (0, 0, -11.4) normal (0, 0, 1) x (1, 0, 0) in component "06 Electronics retaining yoke"
sketch "SPDT keeper pad with 0.35mm axial allowance profile" plane through (0, 0, -11.4) normal (0, 0, 1) x (1, 0, 0) in component "06 Electronics retaining yoke"
  line L0 (37.4, 52) -> (38.6, 52)
  line L1 (38.6, 52) -> (38.6, 54.5)
  line L2 (38.6, 54.5) -> (37.4, 54.5)
  line L3 (37.4, 54.5) -> (37.4, 52)
  dimension "d2029" = 1.2
  dimension "d2030" = 2.5
  measures "d2029" horizontal distance of L0.start L0.end
  measures "d2030" vertical distance of L0.end L1.end
extrude "SPDT keeper pad with 0.35mm axial allowance" add sketch "SPDT keeper pad with 0.35mm axial allowance profile" against normal blind 8.25 separate body makes body 213 in component "06 Electronics retaining yoke"
ref_plane "WorkPlane55" through (0, 0, -11.4) normal (0, 0, 1) x (1, 0, 0) in component "06 Electronics retaining yoke"
sketch "SPDT keeper pad with 0.35mm axial allowance profile (1)" plane through (0, 0, -11.4) normal (0, 0, 1) x (1, 0, 0) in component "06 Electronics retaining yoke"
  line L0 (44.6, 52) -> (45.8, 52)
  line L1 (45.8, 52) -> (45.8, 54.5)
  line L2 (45.8, 54.5) -> (44.6, 54.5)
  line L3 (44.6, 54.5) -> (44.6, 52)
  dimension "d2035" = 1.2
  dimension "d2036" = 2.5
  measures "d2035" horizontal distance of L0.start L0.end
  measures "d2036" vertical distance of L0.end L1.end
extrude "SPDT keeper pad with 0.35mm axial allowance (1)" add sketch "SPDT keeper pad with 0.35mm axial allowance profile (1)" against normal blind 8.25 separate body makes body 214 in component "06 Electronics retaining yoke"
ref_plane "WorkPlane56" through (0, 0, -9.4) normal (0, 0, 1) x (1, 0, 0) in component "06 Electronics retaining yoke"
sketch "SPDT top-opening roof root profile" plane through (0, 0, -9.4) normal (0, 0, 1) x (1, 0, 0) in component "06 Electronics retaining yoke"
  line L0 (37.4, 53) -> (44.6, 53)
  line L1 (44.6, 53) -> (44.6, 59.75)
  line L2 (44.6, 59.75) -> (37.4, 59.75)
  line L3 (37.4, 59.75) -> (37.4, 53)
  dimension "d2041" = 7.2
  dimension "d2042" = 6.75
  measures "d2041" horizontal distance of L0.start L0.end
  measures "d2042" vertical distance of L0.end L1.end
extrude "SPDT top-opening roof root" add sketch "SPDT top-opening roof root profile" against normal blind 2 separate body makes body 215 in component "06 Electronics retaining yoke"
ref_plane "WorkPlane57" through (0, 0, -9.4) normal (0, 0, 1) x (1, 0, 0) in component "06 Electronics retaining yoke"
sketch "SPDT removable lever-slot roof profile" plane through (0, 0, -9.4) normal (0, 0, 1) x (1, 0, 0) in component "06 Electronics retaining yoke"
  line L0 (37.3, 57.3) -> (44.7, 57.3)
  line L1 (44.7, 57.3) -> (44.7, 59.75)
  line L2 (44.7, 59.75) -> (37.3, 59.75)
  line L3 (37.3, 59.75) -> (37.3, 57.3)
  dimension "d2047" = 7.4
  dimension "d2048" = 2.45
  measures "d2047" horizontal distance of L0.start L0.end
  measures "d2048" vertical distance of L0.end L1.end
extrude "SPDT removable lever-slot roof" add sketch "SPDT removable lever-slot roof profile" against normal blind 11.5 separate body makes body 216 in component "06 Electronics retaining yoke"
combine "Union manufactured solid (3)'" operation add target body 106 tool bodies 211 212 213 214 215 216 in component "06 Electronics retaining yoke"
ref_plane "WorkPlane1" through (0, 0, -20) normal (0, 0, 1) x (1, 0, 0) in component "REF SPDT power switch"
sketch "SPDT main body profile" plane through (0, 0, -20) normal (0, 0, 1) x (1, 0, 0) in component "REF SPDT power switch"
  line L0 (35.75, 51.5) -> (46.25, 51.5)
  line L1 (46.25, 51.5) -> (46.25, 57)
  line L2 (46.25, 57) -> (35.75, 57)
  line L3 (35.75, 57) -> (35.75, 51.5)
  dimension "d2053" = 10.5
  dimension "d2054" = 5.5
  measures "d2053" horizontal distance of L0.start L0.end
  measures "d2054" vertical distance of L0.end L1.end
extrude "SPDT main body" add sketch "SPDT main body profile" against normal blind 5.7 separate body makes body 217 in component "REF SPDT power switch"
ref_plane "WorkPlane2" through (0, 0, -20) normal (0, 0, 1) x (1, 0, 0) in component "REF SPDT power switch"
sketch "SPDT flange envelope profile" plane through (0, 0, -20) normal (0, 0, 1) x (1, 0, 0) in component "REF SPDT power switch"
  line L0 (31.25, 56.5) -> (50.75, 56.5)
  line L1 (50.75, 56.5) -> (50.75, 57)
  line L2 (50.75, 57) -> (31.25, 57)
  line L3 (31.25, 57) -> (31.25, 56.5)
  dimension "d2059" = 19.5
  dimension "d2060" = 0.5
  measures "d2059" horizontal distance of L0.start L0.end
  measures "d2060" vertical distance of L0.end L1.end
extrude "SPDT flange envelope" add sketch "SPDT flange envelope profile" against normal blind 5.7 separate body makes body 218 in component "REF SPDT power switch"
ref_plane "WorkPlane3" through (0, 0, -22.55) normal (0, 0, 1) x (1, 0, 0) in component "REF SPDT power switch"
sketch "SPDT solder terminal envelope profile" plane through (0, 0, -22.55) normal (0, 0, 1) x (1, 0, 0) in component "REF SPDT power switch"
  line L0 (36.9, 49) -> (38.1, 49)
  line L1 (38.1, 49) -> (38.1, 51.5)
  line L2 (38.1, 51.5) -> (36.9, 51.5)
  line L3 (36.9, 51.5) -> (36.9, 49)
  dimension "d2065" = 1.2
  dimension "d2066" = 2.5
  measures "d2065" horizontal distance of L0.start L0.end
  measures "d2066" vertical distance of L0.end L1.end
extrude "SPDT solder terminal envelope" add sketch "SPDT solder terminal envelope profile" against normal blind 0.6 separate body makes body 219 in component "REF SPDT power switch"
ref_plane "WorkPlane4" through (0, 0, -22.55) normal (0, 0, 1) x (1, 0, 0) in component "REF SPDT power switch"
sketch "SPDT solder terminal envelope profile (1)" plane through (0, 0, -22.55) normal (0, 0, 1) x (1, 0, 0) in component "REF SPDT power switch"
  line L0 (40.4, 49) -> (41.6, 49)
  line L1 (41.6, 49) -> (41.6, 51.5)
  line L2 (41.6, 51.5) -> (40.4, 51.5)
  line L3 (40.4, 51.5) -> (40.4, 49)
  dimension "d2071" = 1.2
  dimension "d2072" = 2.5
  measures "d2071" horizontal distance of L0.start L0.end
  measures "d2072" vertical distance of L0.end L1.end
extrude "SPDT solder terminal envelope (1)" add sketch "SPDT solder terminal envelope profile (1)" against normal blind 0.6 separate body makes body 220 in component "REF SPDT power switch"
ref_plane "WorkPlane5" through (0, 0, -22.55) normal (0, 0, 1) x (1, 0, 0) in component "REF SPDT power switch"
sketch "SPDT solder terminal envelope profile (2)" plane through (0, 0, -22.55) normal (0, 0, 1) x (1, 0, 0) in component "REF SPDT power switch"
  line L0 (43.9, 49) -> (45.1, 49)
  line L1 (45.1, 49) -> (45.1, 51.5)
  line L2 (45.1, 51.5) -> (43.9, 51.5)
  line L3 (43.9, 51.5) -> (43.9, 49)
  dimension "d2077" = 1.2
  dimension "d2078" = 2.5
  measures "d2077" horizontal distance of L0.start L0.end
  measures "d2078" vertical distance of L0.end L1.end
extrude "SPDT solder terminal envelope (2)" add sketch "SPDT solder terminal envelope profile (2)" against normal blind 0.6 separate body makes body 221 in component "REF SPDT power switch"
ref_plane "WorkPlane1" through (0, 0, -21.25) normal (0, 0, 1) x (1, 0, 0) in component "REF SPDT moving lever"
sketch "SPDT lever profile" plane through (0, 0, -21.25) normal (0, 0, 1) x (1, 0, 0) in component "REF SPDT moving lever"
  line L0 (39.4, 57) -> (42.6, 57)
  line L1 (42.6, 57) -> (42.6, 62)
  line L2 (42.6, 62) -> (39.4, 62)
  line L3 (39.4, 62) -> (39.4, 57)
  dimension "d2083" = 3.2
  dimension "d2084" = 5
  measures "d2083" horizontal distance of L0.start L0.end
  measures "d2084" vertical distance of L0.end L1.end
extrude "SPDT lever" add sketch "SPDT lever profile" against normal blind 3.2 separate body makes body 222 in component "REF SPDT moving lever"
ref_plane "WorkPlane1" through (0, 0, -16.2) normal (0, 0, 1) x (1, 0, 0) in component "REF Capacitor"
sketch "C1 680uF maximum 8x11.5mm profile" plane through (0, 0, -16.2) normal (0, 0, 1) x (1, 0, 0) in component "REF Capacitor"
  circle A0 centre (84, 47.5) radius 4
  dimension "d2089" = 8
  measures "d2089" diameter of A0
extrude "C1 680uF maximum 8x11.5mm" add sketch "C1 680uF maximum 8x11.5mm profile" against normal blind 11.5 separate body makes body 223 in component "REF Capacitor"
component "01 Front optical bezel" placed x (1, 0, 0) y (0, 1, 0) z (0, 0, 1) at (0, 0, 0)
component "02 Clear acrylic" placed x (1, 0, 0) y (0, 1, 0) z (0, 0, 1) at (0, 0, 0)
component "03 Registered graphic backing" placed x (1, 0, 0) y (0, 1, 0) z (0, 0, 1) at (0, 0, 0)
component "04 Optical retainer" placed x (1, 0, 0) y (0, 1, 0) z (0, 0, 1) at (0, 0, 0)
component "81 Laminate front spacer" placed x (1, 0, 0) y (0, 1, 0) z (0, 0, 1) at (0, 0, 0)
component "82 Laminate rear shim" placed x (1, 0, 0) y (0, 1, 0) z (0, 0, 1) at (0, 0, 0)
component "05 Rear electronics housing" placed x (1, 0, 0) y (0, 1, 0) z (0, 0, 1) at (0, 0, 0)
component "06 Electronics retaining yoke" placed x (1, 0, 0) y (0, 1, 0) z (0, 0, 1) at (0, 0, 0)
component "07 Captive reset plunger" placed x (1, 0, 0) y (0, 1, 0) z (0, 0, 1) at (0, 0, 0)
component "08 Captive RUN PROGRAM slider" placed x (1, 0, 0) y (0, 1, 0) z (0, 0, 1) at (0, 0, 0)
component "REF Battery" placed x (1, 0, 0) y (0, 1, 0) z (0, 0, 1) at (0, 0, 0)
component "REF Charger" placed x (1, 0, 0) y (0, 1, 0) z (0, 0, 1) at (0, 0, 0)
component "REF XIAO" placed x (1, 0, 0) y (0, 1, 0) z (0, 0, 1) at (0, 0, 0)
component "REF DPDT" placed x (1, 0, 0) y (0, 1, 0) z (0, 0, 1) at (0, 0, 0)
component "REF Four LEDs" placed x (1, 0, 0) y (0, 1, 0) z (0, 0, 1) at (0, 0, 0)
component "REF M3 screws" placed x (1, 0, 0) y (0, 1, 0) z (0, 0, 1) at (0, 0, 0)
component "REF M3 nuts" placed x (1, 0, 0) y (0, 1, 0) z (0, 0, 1) at (0, 0, 0)
component "REF SPDT power switch" placed x (1, 0, 0) y (0, 1, 0) z (0, 0, 1) at (0, 0, 0)
component "REF SPDT moving lever" placed x (1, 0, 0) y (0, 1, 0) z (0, 0, 1) at (0, 0, 0)
component "REF Capacitor" placed x (1, 0, 0) y (0, 1, 0) z (0, 0, 1) at (0, 0, 0)
equation "case_w = 120.0000000 mm" comment "Front width"